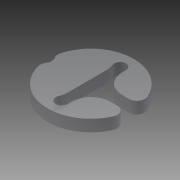
# Autodesk Inventor part: Middle Endcap080813
Saved by Autodesk Inventor 2013 (Build 170138000, 138)
## iProperties
Created: 2013-05-23
Part Number: Middle Endcap080813
Material: Polycarbonate, Clear
Document SubType Name: Modeling
Designer: Eric
Density: 1.2 g/cm^3
Mass: 0.890235 g
Surface Area: 8.2204 cm^2
Volume: 0.741863 cm^3
Author: Eric
Autodesk Inventor part; units mm, degrees
ref_plane "YZ Plane" through (0, 0, 0) normal (1, 0, 0) x (0, 1, 0)
ref_plane "XZ Plane" through (0, 0, 0) normal (0, 1, 0) x (-1, 0, 0)
ref_plane "XY Plane" through (0, 0, 0) normal (0, 0, 1) x (1, 0, 0)
sketch "Sketch1" plane through (0, 0, 0) normal (0, 0, 1) x (1, 0, 0)
  arc A0 (1.4995, 7.5) -> (-1.385, 6.9228) centre (-0.0005, 7.5) ccw
  arc A1 (-1.3846, -6.9231) -> (1.5, -7.5) centre (0, -7.5) ccw
  arc A2 (-10.3524, -1.1528) -> (-10.356, 1.1198) centre (-12, -0.0191) ccw
  arc A3 (10.1341, 4.2778) -> (-10.6479, 2.7607) centre (0, 0) ccw
  arc A4 (-10.6391, -2.7946) -> (10.1341, -4.2778) centre (0, 0) ccw
  arc A5 (-10.6479, 2.7607) -> (-10.356, 1.1198) centre (-8.7119, 2.2588) ccw
  arc A6 (-10.3524, -1.1528) -> (-10.6391, -2.7946) centre (-8.7047, -2.2865) ccw
  line L0 (-1, -5) -> (-1, 4.9988)
  arc A7 (-1, 4.9988) -> (-1.385, 6.9228) centre (-6, 4.9988) ccw
  arc A8 (-1.3846, -6.9231) -> (-1, -5) centre (-6, -5) ccw
  line L1 (1.4995, 7.5) -> (1.4995, 6.5)
  line L2 (1.4995, -6.5) -> (1.4995, -7.5382)
  line L3 (6.4995, -1.5) -> (8.2916, -1.5)
  line L4 (6.4995, 1.5) -> (8.2916, 1.5)
  arc A9 (6.4995, -1.5) -> (1.4995, -6.5) centre (6.4995, -6.5) ccw
  arc A10 (1.4995, 6.5) -> (6.4995, 1.5) centre (6.4995, 6.5) ccw
  arc A11 (10.1341, -4.2778) -> (8.2916, -1.5) centre (8.2916, -3.5) ccw
  arc A12 (8.2916, 1.5) -> (10.1341, 4.2778) centre (8.2916, 3.5) ccw
  point P0 (10.8972, -1.5)
  point P1 (10.8972, 1.5)
  point P2 (1.4995, 1.5)
  point P3 (1.4995, -1.5)
  point P4 (-1, -6.382)
  point P5 (-1, 6.3815)
  dimension "d5" = 3
  dimension "d6" = 3
  dimension "d7" = 15
  dimension "d18" = 7.5
  dimension "d20" = 4
  dimension "d21" = 12
  dimension "d22" = 2
  dimension "d26" = 5
  dimension "d27" = 5
  dimension "d28" = 2
  constraints: 31 point on circle, 18 tangent, 13 centre point, 10 end point, 8 point on line, 4 equal radius, 1 coincident, 1 parallel, 1 perpendicular
  measures "d5" diameter of A0
  measures "d6" diameter of A1
  measures "d7" distance of A1.centre A0.centre
  measures "d18" distance of point (0, 0) A0.centre
  measures "d20" diameter of A2
  measures "d21" distance of point (0, 0) A2.centre
  measures "d22" radius of A5
  measures "d26" radius of A7
  measures "d27" radius of A9
  measures "d28" radius of A11
extrude "Extrusion2" add sketch "Sketch1" along normal blind 3
body "Solid2"
